Autodesk Fusion 360 part; units mm, degrees
(part 2 of 3)
sketch "b bottom circles" plane through (0, 0, 0) normal (0, 0, 1) x (1, 0, 0) in component "b bottom component"
  line L0 (152.01, 0) -> (302.01, 0)
  line L1 (302.01, 0) -> (302.01, 120)
  line L2 (302.01, 120) -> (152.01, 120)
  line L3 (152.01, 120) -> (152.01, 0)
  circle A0 centre (162.7006, 2.3644) radius 1.005
  circle A1 centre (171.3194, 2.3644) radius 1.005
  circle A2 centre (182.7006, 2.3644) radius 1.005
  circle A3 centre (191.3194, 2.3644) radius 1.005
  circle A4 centre (202.7006, 2.3644) radius 1.005
  circle A5 centre (211.3194, 2.3644) radius 1.005
  circle A6 centre (222.7006, 2.3644) radius 1.005
  circle A7 centre (231.3194, 2.3644) radius 1.005
  circle A8 centre (242.7006, 2.3644) radius 1.005
  circle A9 centre (251.3194, 2.3644) radius 1.005
  circle A10 centre (262.7006, 2.3644) radius 1.005
  circle A11 centre (271.3194, 2.3644) radius 1.005
  circle A12 centre (282.7006, 2.3644) radius 1.005
  circle A13 centre (291.3194, 2.3644) radius 1.005
  circle A14 centre (299.6456, 15.6906) radius 1.005
  circle A15 centre (299.6456, 24.3094) radius 1.005
  circle A16 centre (299.6456, 35.6906) radius 1.005
  circle A17 centre (299.6456, 44.3094) radius 1.005
  circle A18 centre (299.6456, 55.6906) radius 1.005
  circle A19 centre (299.6456, 64.3094) radius 1.005
  circle A20 centre (299.6456, 75.6906) radius 1.005
  circle A21 centre (299.6456, 84.3094) radius 1.005
  circle A22 centre (299.6456, 95.6906) radius 1.005
  circle A23 centre (299.6456, 104.3094) radius 1.005
  circle A24 centre (162.7006, 117.6356) radius 1.005
  circle A25 centre (171.3194, 117.6356) radius 1.005
  circle A26 centre (182.7006, 117.6356) radius 1.005
  circle A27 centre (191.3194, 117.6356) radius 1.005
  circle A28 centre (202.7006, 117.6356) radius 1.005
  circle A29 centre (211.3194, 117.6356) radius 1.005
  circle A30 centre (222.7006, 117.6356) radius 1.005
  circle A31 centre (231.3194, 117.6356) radius 1.005
  circle A32 centre (242.7006, 117.6356) radius 1.005
  circle A33 centre (251.3194, 117.6356) radius 1.005
  circle A34 centre (262.7006, 117.6356) radius 1.005
  circle A35 centre (271.3194, 117.6356) radius 1.005
  circle A36 centre (282.7006, 117.6356) radius 1.005
  circle A37 centre (291.3194, 117.6356) radius 1.005
  circle A38 centre (154.3744, 15.6906) radius 1.005
  circle A39 centre (154.3744, 24.3094) radius 1.005
  circle A40 centre (154.3744, 35.6906) radius 1.005
  circle A41 centre (154.3744, 44.3094) radius 1.005
  circle A42 centre (154.3744, 55.6906) radius 1.005
  circle A43 centre (154.3744, 64.3094) radius 1.005
  circle A44 centre (154.3744, 75.6906) radius 1.005
  circle A45 centre (154.3744, 84.3094) radius 1.005
  circle A46 centre (154.3744, 95.6906) radius 1.005
  circle A47 centre (154.3744, 104.3094) radius 1.005
  dimension "d1612" = 2.01
  dimension "d1613" = 2.01
  dimension "d1614" = 2.01
  dimension "d1615" = 2.01
  dimension "d1616" = 2.01
  dimension "d1617" = 2.01
  dimension "d1618" = 2.01
  dimension "d1619" = 2.01
  dimension "d1620" = 2.01
  dimension "d1621" = 2.01
  dimension "d1622" = 2.01
  dimension "d1623" = 2.01
  dimension "d1624" = 2.01
  dimension "d1625" = 2.01
  dimension "d1647" = 2.01
  dimension "d1648" = 2.01
  dimension "d1649" = 2.01
  dimension "d1650" = 2.01
  dimension "d1651" = 2.01
  dimension "d1652" = 2.01
  dimension "d1653" = 2.01
  dimension "d1654" = 2.01
  dimension "d1655" = 2.01
  dimension "d1656" = 2.01
  dimension "d1686" = 2.01
  dimension "d1687" = 2.01
  dimension "d1688" = 2.01
  dimension "d1689" = 2.01
  dimension "d1690" = 2.01
  dimension "d1691" = 2.01
  dimension "d1692" = 2.01
  dimension "d1693" = 2.01
  dimension "d1694" = 2.01
  dimension "d1695" = 2.01
  dimension "d1696" = 2.01
  dimension "d1697" = 2.01
  dimension "d1698" = 2.01
  dimension "d1699" = 2.01
  dimension "d1721" = 2.01
  dimension "d1722" = 2.01
  dimension "d1723" = 2.01
  dimension "d1724" = 2.01
  dimension "d1725" = 2.01
  dimension "d1726" = 2.01
  dimension "d1727" = 2.01
  dimension "d1728" = 2.01
  dimension "d1729" = 2.01
  dimension "d1730" = 2.01
  measures "d1612" diameter of A0
  measures "d1613" diameter of A1
  measures "d1614" diameter of A2
  measures "d1615" diameter of A3
  measures "d1616" diameter of A4
  measures "d1617" diameter of A5
  measures "d1618" diameter of A6
  measures "d1619" diameter of A7
  measures "d1620" diameter of A8
  measures "d1621" diameter of A9
  measures "d1622" diameter of A10
  measures "d1623" diameter of A11
  measures "d1624" diameter of A12
  measures "d1625" diameter of A13
  measures "d1647" diameter of A14
  measures "d1648" diameter of A15
  measures "d1649" diameter of A16
  measures "d1650" diameter of A17
  measures "d1651" diameter of A18
  measures "d1652" diameter of A19
  measures "d1653" diameter of A20
  measures "d1654" diameter of A21
  measures "d1655" diameter of A22
  measures "d1656" diameter of A23
  measures "d1686" diameter of A24
  measures "d1687" diameter of A25
  measures "d1688" diameter of A26
  measures "d1689" diameter of A27
  measures "d1690" diameter of A28
  measures "d1691" diameter of A29
  measures "d1692" diameter of A30
  measures "d1693" diameter of A31
  measures "d1694" diameter of A32
  measures "d1695" diameter of A33
  measures "d1696" diameter of A34
  measures "d1697" diameter of A35
  measures "d1698" diameter of A36
  measures "d1699" diameter of A37
  measures "d1721" diameter of A38
  measures "d1722" diameter of A39
  measures "d1723" diameter of A40
  measures "d1724" diameter of A41
  measures "d1725" diameter of A42
  measures "d1726" diameter of A43
  measures "d1727" diameter of A44
  measures "d1728" diameter of A45
  measures "d1729" diameter of A46
  measures "d1730" diameter of A47
extrude "b bottom lines body extrude" add sketch "b bottom lines" along normal blind 3.175 separate body makes body 4 in component "b bottom component"
extrude "b bottom circles extrude" add sketch "b bottom circles" along normal blind 3.175 separate body makes body 5 in component "b bottom component"
combine "b bottom lines final combine feature" operation intersect target body 4 tool bodies 5 in component "b bottom component"
sketch "b front lines" plane through (0, 0, 0) normal (0, 0, 1) x (1, 0, 0) in component "b front component"
  line L0 (3.175, 125.185) -> (9.9, 125.185)
  line L1 (9.9, 125.185) -> (9.9, 122.01)
  line L2 (9.9, 122.01) -> (20.1, 122.01)
  line L3 (20.1, 122.01) -> (20.1, 125.185)
  line L4 (20.1, 125.185) -> (29.9, 125.185)
  line L5 (29.9, 125.185) -> (29.9, 122.01)
  line L6 (29.9, 122.01) -> (40.1, 122.01)
  line L7 (40.1, 122.01) -> (40.1, 125.185)
  line L8 (40.1, 125.185) -> (46.825, 125.185)
  line L9 (46.825, 125.185) -> (46.825, 131.91)
  line L10 (46.825, 131.91) -> (50, 131.91)
  line L11 (50, 131.91) -> (50, 142.11)
  line L12 (50, 142.11) -> (46.825, 142.11)
  line L13 (46.825, 142.11) -> (46.825, 151.91)
  line L14 (46.825, 151.91) -> (50, 151.91)
  line L15 (50, 151.91) -> (50, 162.11)
  line L16 (50, 162.11) -> (46.825, 162.11)
  line L17 (46.825, 162.11) -> (46.825, 171.91)
  line L18 (46.825, 171.91) -> (50, 171.91)
  line L19 (50, 171.91) -> (50, 182.11)
  line L20 (50, 182.11) -> (46.825, 182.11)
  line L21 (46.825, 182.11) -> (46.825, 191.91)
  line L22 (46.825, 191.91) -> (50, 191.91)
  line L23 (50, 191.91) -> (50, 202.11)
  line L24 (50, 202.11) -> (46.825, 202.11)
  line L25 (46.825, 202.11) -> (46.825, 211.91)
  line L26 (46.825, 211.91) -> (50, 211.91)
  line L27 (50, 211.91) -> (50, 222.11)
  line L28 (50, 222.11) -> (46.825, 222.11)
  line L29 (46.825, 222.11) -> (46.825, 231.91)
  line L30 (46.825, 231.91) -> (50, 231.91)
  line L31 (50, 231.91) -> (50, 242.11)
  line L32 (50, 242.11) -> (46.825, 242.11)
  line L33 (46.825, 242.11) -> (46.825, 251.91)
  line L34 (46.825, 251.91) -> (50, 251.91)
  line L35 (50, 251.91) -> (50, 262.11)
  line L36 (50, 262.11) -> (46.825, 262.11)
  line L37 (46.825, 262.11) -> (46.825, 268.835)
  line L38 (3.175, 268.835) -> (9.9, 268.835)
  line L39 (9.9, 268.835) -> (9.9, 272.01)
  line L40 (9.9, 272.01) -> (20.1, 272.01)
  line L41 (20.1, 272.01) -> (20.1, 268.835)
  line L42 (20.1, 268.835) -> (29.9, 268.835)
  line L43 (29.9, 268.835) -> (29.9, 272.01)
  line L44 (29.9, 272.01) -> (40.1, 272.01)
  line L45 (40.1, 272.01) -> (40.1, 268.835)
  line L46 (40.1, 268.835) -> (46.825, 268.835)
  line L47 (3.175, 125.185) -> (3.175, 131.91)
  line L48 (3.175, 131.91) -> (0, 131.91)
  line L49 (0, 131.91) -> (0, 142.11)
  line L50 (0, 142.11) -> (3.175, 142.11)
  line L51 (3.175, 142.11) -> (3.175, 151.91)
  line L52 (3.175, 151.91) -> (0, 151.91)
  line L53 (0, 151.91) -> (0, 162.11)
  line L54 (0, 162.11) -> (3.175, 162.11)
  line L55 (3.175, 162.11) -> (3.175, 171.91)
  line L56 (3.175, 171.91) -> (0, 171.91)
  line L57 (0, 171.91) -> (0, 182.11)
  line L58 (0, 182.11) -> (3.175, 182.11)
  line L59 (3.175, 182.11) -> (3.175, 191.91)
  line L60 (3.175, 191.91) -> (0, 191.91)
  line L61 (0, 191.91) -> (0, 202.11)
  line L62 (0, 202.11) -> (3.175, 202.11)
  line L63 (3.175, 202.11) -> (3.175, 211.91)
  line L64 (3.175, 211.91) -> (0, 211.91)
  line L65 (0, 211.91) -> (0, 222.11)
  line L66 (0, 222.11) -> (3.175, 222.11)
  line L67 (3.175, 222.11) -> (3.175, 231.91)
  line L68 (3.175, 231.91) -> (0, 231.91)
  line L69 (0, 231.91) -> (0, 242.11)
  line L70 (0, 242.11) -> (3.175, 242.11)
  line L71 (3.175, 242.11) -> (3.175, 251.91)
  line L72 (3.175, 251.91) -> (0, 251.91)
  line L73 (0, 251.91) -> (0, 262.11)
  line L74 (0, 262.11) -> (3.175, 262.11)
  line L75 (3.175, 262.11) -> (3.175, 268.835)
  dimension "d1735" = 6.725
  dimension "d1736" = 3.175
  dimension "d1737" = 10.2
  dimension "d1738" = 3.175
  dimension "d1739" = 9.8
  dimension "d1740" = 3.175
  dimension "d1741" = 10.2
  dimension "d1742" = 3.175
  dimension "d1743" = 6.725
  dimension "d1748" = 6.725
  dimension "d1749" = 3.175
  dimension "d1750" = 10.2
  dimension "d1751" = 3.175
  dimension "d1752" = 9.8
  dimension "d1753" = 3.175
  dimension "d1754" = 10.2
  dimension "d1755" = 3.175
  dimension "d1756" = 9.8
  dimension "d1757" = 3.175
  dimension "d1758" = 10.2
  dimension "d1759" = 3.175
  dimension "d1760" = 9.8
  dimension "d1761" = 3.175
  dimension "d1762" = 10.2
  dimension "d1763" = 3.175
  dimension "d1764" = 9.8
  dimension "d1765" = 3.175
  dimension "d1766" = 10.2
  dimension "d1767" = 3.175
  dimension "d1768" = 9.8
  dimension "d1769" = 3.175
  dimension "d1770" = 10.2
  dimension "d1771" = 3.175
  dimension "d1772" = 9.8
  dimension "d1773" = 3.175
  dimension "d1774" = 10.2
  dimension "d1775" = 3.175
  dimension "d1776" = 6.725
  dimension "d1791" = 6.725
  dimension "d1792" = 3.175
  dimension "d1793" = 10.2
  dimension "d1794" = 3.175
  dimension "d1795" = 9.8
  dimension "d1796" = 3.175
  dimension "d1797" = 10.2
  dimension "d1798" = 3.175
  dimension "d1799" = 6.725
  dimension "d1804" = 6.725
  dimension "d1805" = 3.175
  dimension "d1806" = 10.2
  dimension "d1807" = 3.175
  dimension "d1808" = 9.8
  dimension "d1809" = 3.175
  dimension "d1810" = 10.2
  dimension "d1811" = 3.175
  dimension "d1812" = 9.8
  dimension "d1813" = 3.175
  dimension "d1814" = 10.2
  dimension "d1815" = 3.175
  dimension "d1816" = 9.8
  dimension "d1817" = 3.175
  dimension "d1818" = 10.2
  dimension "d1819" = 3.175
  dimension "d1820" = 9.8
  dimension "d1821" = 3.175
  dimension "d1822" = 10.2
  dimension "d1823" = 3.175
  dimension "d1824" = 9.8
  dimension "d1825" = 3.175
  dimension "d1826" = 10.2
  dimension "d1827" = 3.175
  dimension "d1828" = 9.8
  dimension "d1829" = 3.175
  dimension "d1830" = 10.2
  dimension "d1831" = 3.175
  dimension "d1832" = 6.725
  constraint horizontal L0
  constraint vertical L1
  constraint horizontal L2
  constraint vertical L3
  constraint horizontal L4
  constraint vertical L5
  constraint horizontal L6
  constraint vertical L7
  constraint horizontal L8
  constraint vertical L9
  constraint horizontal L10
  constraint vertical L11
  constraint horizontal L12
  constraint vertical L13
  constraint horizontal L14
  constraint vertical L15
  constraint horizontal L16
  constraint vertical L17
  constraint horizontal L18
  constraint vertical L19
  constraint horizontal L20
  constraint vertical L21
  constraint horizontal L22
  constraint vertical L23
  constraint horizontal L24
  constraint vertical L25
  constraint horizontal L26
  constraint vertical L27
  constraint horizontal L28
  constraint vertical L29
  constraint horizontal L30
  constraint vertical L31
  constraint horizontal L32
  constraint vertical L33
  constraint horizontal L34
  constraint vertical L35
  constraint horizontal L36
  constraint vertical L37
  constraint horizontal L38
  constraint vertical L39
  constraint horizontal L40
  constraint vertical L41
  constraint horizontal L42
  constraint vertical L43
  constraint horizontal L44
  constraint vertical L45
  constraint horizontal L46
  constraint vertical L47
  constraint horizontal L48
  constraint vertical L49
  constraint horizontal L50
  constraint vertical L51
  constraint horizontal L52
  constraint vertical L53
  constraint horizontal L54
  constraint vertical L55
  constraint horizontal L56
  constraint vertical L57
  constraint horizontal L58
  constraint vertical L59
  constraint horizontal L60
  constraint vertical L61
  constraint horizontal L62
  constraint vertical L63
  constraint horizontal L64
  constraint vertical L65
  constraint horizontal L66
  constraint vertical L67
  constraint horizontal L68
  constraint vertical L69
  constraint horizontal L70
  constraint vertical L71
  constraint horizontal L72
  constraint vertical L73
  constraint horizontal L74
  constraint vertical L75
  measures "d1735" distance of L0.start L0.end
  measures "d1736" distance of L0.end L1.end
  measures "d1737" distance of L1.end L2.end
  measures "d1738" distance of L2.end L3.end
  measures "d1739" distance of L3.end L4.end
  measures "d1740" distance of L4.end L5.end
  measures "d1741" distance of L5.end L6.end
  measures "d1742" distance of L6.end L7.end
  measures "d1743" distance of L7.end L8.end
  measures "d1748" distance of L8.end L9.end
  measures "d1749" distance of L9.end L10.end
  measures "d1750" distance of L10.end L11.end
  measures "d1751" distance of L11.end L12.end
  measures "d1752" distance of L12.end L13.end
  measures "d1753" distance of L13.end L14.end
  measures "d1754" distance of L14.end L15.end
  measures "d1755" distance of L15.end L16.end
  measures "d1756" distance of L16.end L17.end
  measures "d1757" distance of L17.end L18.end
  measures "d1758" distance of L18.end L19.end
  measures "d1759" distance of L19.end L20.end
  measures "d1760" distance of L20.end L21.end
  measures "d1761" distance of L21.end L22.end
  measures "d1762" distance of L22.end L23.end
  measures "d1763" distance of L23.end L24.end
  measures "d1764" distance of L24.end L25.end
  measures "d1765" distance of L25.end L26.end
  measures "d1766" distance of L26.end L27.end
  measures "d1767" distance of L27.end L28.end
  measures "d1768" distance of L28.end L29.end
  measures "d1769" distance of L29.end L30.end
  measures "d1770" distance of L30.end L31.end
  measures "d1771" distance of L31.end L32.end
  measures "d1772" distance of L32.end L33.end
  measures "d1773" distance of L33.end L34.end
  measures "d1774" distance of L34.end L35.end
  measures "d1775" distance of L35.end L36.end
  measures "d1776" distance of L36.end L37.end
  measures "d1791" distance of L38.start L38.end
  measures "d1792" distance of L38.end L39.end
  measures "d1793" distance of L39.end L40.end
  measures "d1794" distance of L40.end L41.end
  measures "d1795" distance of L41.end L42.end
  measures "d1796" distance of L42.end L43.end
  measures "d1797" distance of L43.end L44.end
  measures "d1798" distance of L44.end L45.end
  measures "d1799" distance of L37.end L45.end
  measures "d1804" distance of L0.start L47.end
  measures "d1805" distance of L47.end L48.end
  measures "d1806" distance of L48.end L49.end
  measures "d1807" distance of L49.end L50.end
  measures "d1808" distance of L50.end L51.end
  measures "d1809" distance of L51.end L52.end
  measures "d1810" distance of L52.end L53.end
  measures "d1811" distance of L53.end L54.end
  measures "d1812" distance of L54.end L55.end
  measures "d1813" distance of L55.end L56.end
  measures "d1814" distance of L56.end L57.end
  measures "d1815" distance of L57.end L58.end
  measures "d1816" distance of L58.end L59.end
  measures "d1817" distance of L59.end L60.end
  measures "d1818" distance of L60.end L61.end
  measures "d1819" distance of L61.end L62.end
  measures "d1820" distance of L62.end L63.end
  measures "d1821" distance of L63.end L64.end
  measures "d1822" distance of L64.end L65.end
  measures "d1823" distance of L65.end L66.end
  measures "d1824" distance of L66.end L67.end
  measures "d1825" distance of L67.end L68.end
  measures "d1826" distance of L68.end L69.end
  measures "d1827" distance of L69.end L70.end
  measures "d1828" distance of L70.end L71.end
  measures "d1829" distance of L71.end L72.end
  measures "d1830" distance of L72.end L73.end
  measures "d1831" distance of L73.end L74.end
  measures "d1832" distance of L38.start L74.end
sketch "b front circles" plane through (0, 0, 0) normal (0, 0, 1) x (1, 0, 0) in component "b front component"
  line L0 (0, 122.01) -> (50, 122.01)
  line L1 (50, 122.01) -> (50, 272.01)
  line L2 (50, 272.01) -> (0, 272.01)
  line L3 (0, 272.01) -> (0, 122.01)
  circle A0 centre (9.3094, 124.3744) radius 1.005
  circle A1 centre (20.6906, 124.3744) radius 1.005
  circle A2 centre (29.3094, 124.3744) radius 1.005
  circle A3 centre (40.6906, 124.3744) radius 1.005
  circle A4 centre (47.6356, 131.3194) radius 1.005
  circle A5 centre (47.6356, 142.7006) radius 1.005
  circle A6 centre (47.6356, 151.3194) radius 1.005
  circle A7 centre (47.6356, 162.7006) radius 1.005
  circle A8 centre (47.6356, 171.3194) radius 1.005
  circle A9 centre (47.6356, 182.7006) radius 1.005
  circle A10 centre (47.6356, 191.3194) radius 1.005
  circle A11 centre (47.6356, 202.7006) radius 1.005
  circle A12 centre (47.6356, 211.3194) radius 1.005
  circle A13 centre (47.6356, 222.7006) radius 1.005
  circle A14 centre (47.6356, 231.3194) radius 1.005
  circle A15 centre (47.6356, 242.7006) radius 1.005
  circle A16 centre (47.6356, 251.3194) radius 1.005
  circle A17 centre (47.6356, 262.7006) radius 1.005
  circle A18 centre (9.3094, 269.6456) radius 1.005
  circle A19 centre (20.6906, 269.6456) radius 1.005
  circle A20 centre (29.3094, 269.6456) radius 1.005
  circle A21 centre (40.6906, 269.6456) radius 1.005
  circle A22 centre (2.3644, 131.3194) radius 1.005
  circle A23 centre (2.3644, 142.7006) radius 1.005
  circle A24 centre (2.3644, 151.3194) radius 1.005
  circle A25 centre (2.3644, 162.7006) radius 1.005
  circle A26 centre (2.3644, 171.3194) radius 1.005
  circle A27 centre (2.3644, 182.7006) radius 1.005
  circle A28 centre (2.3644, 191.3194) radius 1.005
  circle A29 centre (2.3644, 202.7006) radius 1.005
  circle A30 centre (2.3644, 211.3194) radius 1.005
  circle A31 centre (2.3644, 222.7006) radius 1.005
  circle A32 centre (2.3644, 231.3194) radius 1.005
  circle A33 centre (2.3644, 242.7006) radius 1.005
  circle A34 centre (2.3644, 251.3194) radius 1.005
  circle A35 centre (2.3644, 262.7006) radius 1.005
  dimension "d1744" = 2.01
  dimension "d1745" = 2.01
  dimension "d1746" = 2.01
  dimension "d1747" = 2.01
  dimension "d1777" = 2.01
  dimension "d1778" = 2.01
  dimension "d1779" = 2.01
  dimension "d1780" = 2.01
  dimension "d1781" = 2.01
  dimension "d1782" = 2.01
  dimension "d1783" = 2.01
  dimension "d1784" = 2.01
  dimension "d1785" = 2.01
  dimension "d1786" = 2.01
  dimension "d1787" = 2.01
  dimension "d1788" = 2.01
  dimension "d1789" = 2.01
  dimension "d1790" = 2.01
  dimension "d1800" = 2.01
  dimension "d1801" = 2.01
  dimension "d1802" = 2.01
  dimension "d1803" = 2.01
  dimension "d1833" = 2.01
  dimension "d1834" = 2.01
  dimension "d1835" = 2.01
  dimension "d1836" = 2.01
  dimension "d1837" = 2.01
  dimension "d1838" = 2.01
  dimension "d1839" = 2.01
  dimension "d1840" = 2.01
  dimension "d1841" = 2.01
  dimension "d1842" = 2.01
  dimension "d1843" = 2.01
  dimension "d1844" = 2.01
  dimension "d1845" = 2.01
  dimension "d1846" = 2.01
  measures "d1744" diameter of A0
  measures "d1745" diameter of A1
  measures "d1746" diameter of A2
  measures "d1747" diameter of A3
  measures "d1777" diameter of A4
  measures "d1778" diameter of A5
  measures "d1779" diameter of A6
  measures "d1780" diameter of A7
  measures "d1781" diameter of A8
  measures "d1782" diameter of A9
  measures "d1783" diameter of A10
  measures "d1784" diameter of A11
  measures "d1785" diameter of A12
  measures "d1786" diameter of A13
  measures "d1787" diameter of A14
  measures "d1788" diameter of A15
  measures "d1789" diameter of A16
  measures "d1790" diameter of A17
  measures "d1800" diameter of A18
  measures "d1801" diameter of A19
  measures "d1802" diameter of A20
  measures "d1803" diameter of A21
  measures "d1833" diameter of A22
  measures "d1834" diameter of A23
  measures "d1835" diameter of A24
  measures "d1836" diameter of A25
  measures "d1837" diameter of A26
  measures "d1838" diameter of A27
  measures "d1839" diameter of A28
  measures "d1840" diameter of A29
  measures "d1841" diameter of A30
  measures "d1842" diameter of A31
  measures "d1843" diameter of A32
  measures "d1844" diameter of A33
  measures "d1845" diameter of A34
  measures "d1846" diameter of A35
extrude "b front lines body extrude" add sketch "b front lines" along normal blind 3.175 separate body makes body 6 in component "b front component"
extrude "b front circles extrude" add sketch "b front circles" along normal blind 3.175 separate body makes body 7 in component "b front component"
combine "b front lines final combine feature" operation intersect target body 6 tool bodies 7 in component "b front component"
sketch "b back lines" plane through (0, 0, 0) normal (0, 0, 1) x (1, 0, 0) in component "b back component"
  line L0 (55.185, 125.185) -> (61.91, 125.185)
  line L1 (61.91, 125.185) -> (61.91, 122.01)
  line L2 (61.91, 122.01) -> (72.11, 122.01)
  line L3 (72.11, 122.01) -> (72.11, 125.185)
  line L4 (72.11, 125.185) -> (81.91, 125.185)
  line L5 (81.91, 125.185) -> (81.91, 122.01)
  line L6 (81.91, 122.01) -> (92.11, 122.01)
  line L7 (92.11, 122.01) -> (92.11, 125.185)
  line L8 (92.11, 125.185) -> (98.835, 125.185)
  line L9 (98.835, 125.185) -> (98.835, 131.91)
  line L10 (98.835, 131.91) -> (102.01, 131.91)
  line L11 (102.01, 131.91) -> (102.01, 142.11)
  line L12 (102.01, 142.11) -> (98.835, 142.11)
  line L13 (98.835, 142.11) -> (98.835, 151.91)
  line L14 (98.835, 151.91) -> (102.01, 151.91)
  line L15 (102.01, 151.91) -> (102.01, 162.11)
  line L16 (102.01, 162.11) -> (98.835, 162.11)
  line L17 (98.835, 162.11) -> (98.835, 171.91)
  line L18 (98.835, 171.91) -> (102.01, 171.91)
  line L19 (102.01, 171.91) -> (102.01, 182.11)
  line L20 (102.01, 182.11) -> (98.835, 182.11)
  line L21 (98.835, 182.11) -> (98.835, 191.91)
  line L22 (98.835, 191.91) -> (102.01, 191.91)
  line L23 (102.01, 191.91) -> (102.01, 202.11)
  line L24 (102.01, 202.11) -> (98.835, 202.11)
  line L25 (98.835, 202.11) -> (98.835, 211.91)
  line L26 (98.835, 211.91) -> (102.01, 211.91)
  line L27 (102.01, 211.91) -> (102.01, 222.11)
  line L28 (102.01, 222.11) -> (98.835, 222.11)
  line L29 (98.835, 222.11) -> (98.835, 231.91)
  line L30 (98.835, 231.91) -> (102.01, 231.91)
  line L31 (102.01, 231.91) -> (102.01, 242.11)
  line L32 (102.01, 242.11) -> (98.835, 242.11)
  line L33 (98.835, 242.11) -> (98.835, 251.91)
  line L34 (98.835, 251.91) -> (102.01, 251.91)
  line L35 (102.01, 251.91) -> (102.01, 262.11)
  line L36 (102.01, 262.11) -> (98.835, 262.11)
  line L37 (98.835, 262.11) -> (98.835, 268.835)
  line L38 (55.185, 268.835) -> (61.91, 268.835)
  line L39 (61.91, 268.835) -> (61.91, 272.01)
  line L40 (61.91, 272.01) -> (72.11, 272.01)
  line L41 (72.11, 272.01) -> (72.11, 268.835)
  line L42 (72.11, 268.835) -> (81.91, 268.835)
  line L43 (81.91, 268.835) -> (81.91, 272.01)
  line L44 (81.91, 272.01) -> (92.11, 272.01)
  line L45 (92.11, 272.01) -> (92.11, 268.835)
  line L46 (92.11, 268.835) -> (98.835, 268.835)
  line L47 (55.185, 125.185) -> (55.185, 131.91)
  line L48 (55.185, 131.91) -> (52.01, 131.91)
  line L49 (52.01, 131.91) -> (52.01, 142.11)
  line L50 (52.01, 142.11) -> (55.185, 142.11)
  line L51 (55.185, 142.11) -> (55.185, 151.91)
  line L52 (55.185, 151.91) -> (52.01, 151.91)
  line L53 (52.01, 151.91) -> (52.01, 162.11)
  line L54 (52.01, 162.11) -> (55.185, 162.11)
  line L55 (55.185, 162.11) -> (55.185, 171.91)
  line L56 (55.185, 171.91) -> (52.01, 171.91)
  line L57 (52.01, 171.91) -> (52.01, 182.11)
  line L58 (52.01, 182.11) -> (55.185, 182.11)
  line L59 (55.185, 182.11) -> (55.185, 191.91)
  line L60 (55.185, 191.91) -> (52.01, 191.91)
  line L61 (52.01, 191.91) -> (52.01, 202.11)
  line L62 (52.01, 202.11) -> (55.185, 202.11)
  line L63 (55.185, 202.11) -> (55.185, 211.91)
  line L64 (55.185, 211.91) -> (52.01, 211.91)
  line L65 (52.01, 211.91) -> (52.01, 222.11)
  line L66 (52.01, 222.11) -> (55.185, 222.11)
  line L67 (55.185, 222.11) -> (55.185, 231.91)
  line L68 (55.185, 231.91) -> (52.01, 231.91)
  line L69 (52.01, 231.91) -> (52.01, 242.11)
  line L70 (52.01, 242.11) -> (55.185, 242.11)
  line L71 (55.185, 242.11) -> (55.185, 251.91)
  line L72 (55.185, 251.91) -> (52.01, 251.91)
  line L73 (52.01, 251.91) -> (52.01, 262.11)
  line L74 (52.01, 262.11) -> (55.185, 262.11)
  line L75 (55.185, 262.11) -> (55.185, 268.835)
  dimension "d1851" = 6.725
  dimension "d1852" = 3.175
  dimension "d1853" = 10.2
  dimension "d1854" = 3.175
  dimension "d1855" = 9.8
  dimension "d1856" = 3.175
  dimension "d1857" = 10.2
  dimension "d1858" = 3.175
  dimension "d1859" = 6.725
  dimension "d1864" = 6.725
  dimension "d1865" = 3.175
  dimension "d1866" = 10.2
  dimension "d1867" = 3.175
  dimension "d1868" = 9.8
  dimension "d1869" = 3.175
  dimension "d1870" = 10.2
  dimension "d1871" = 3.175
  dimension "d1872" = 9.8
  dimension "d1873" = 3.175
  dimension "d1874" = 10.2
  dimension "d1875" = 3.175
  dimension "d1876" = 9.8
  dimension "d1877" = 3.175
  dimension "d1878" = 10.2
  dimension "d1879" = 3.175
  dimension "d1880" = 9.8
  dimension "d1881" = 3.175
  dimension "d1882" = 10.2
  dimension "d1883" = 3.175
  dimension "d1884" = 9.8
  dimension "d1885" = 3.175
  dimension "d1886" = 10.2
  dimension "d1887" = 3.175
  dimension "d1888" = 9.8
  dimension "d1889" = 3.175
  dimension "d1890" = 10.2
  dimension "d1891" = 3.175
  dimension "d1892" = 6.725
  dimension "d1907" = 6.725
  dimension "d1908" = 3.175
  dimension "d1909" = 10.2
  dimension "d1910" = 3.175
  dimension "d1911" = 9.8
  dimension "d1912" = 3.175
  dimension "d1913" = 10.2
  dimension "d1914" = 3.175
  dimension "d1915" = 6.725
  dimension "d1920" = 6.725
  dimension "d1921" = 3.175
  dimension "d1922" = 10.2
  dimension "d1923" = 3.175
  dimension "d1924" = 9.8
  dimension "d1925" = 3.175
  dimension "d1926" = 10.2
  dimension "d1927" = 3.175
  dimension "d1928" = 9.8
  dimension "d1929" = 3.175
  dimension "d1930" = 10.2
  dimension "d1931" = 3.175
  dimension "d1932" = 9.8
  dimension "d1933" = 3.175
  dimension "d1934" = 10.2
  dimension "d1935" = 3.175
  dimension "d1936" = 9.8
  dimension "d1937" = 3.175
  dimension "d1938" = 10.2
  dimension "d1939" = 3.175
  dimension "d1940" = 9.8
  dimension "d1941" = 3.175
  dimension "d1942" = 10.2
  dimension "d1943" = 3.175
  dimension "d1944" = 9.8
  dimension "d1945" = 3.175
  dimension "d1946" = 10.2
  dimension "d1947" = 3.175
  dimension "d1948" = 6.725
  constraint horizontal L0
  constraint vertical L1
  constraint horizontal L2
  constraint vertical L3
  constraint horizontal L4
  constraint vertical L5
  constraint horizontal L6
  constraint vertical L7
  constraint horizontal L8
  constraint vertical L9
  constraint horizontal L10
  constraint vertical L11
  constraint horizontal L12
  constraint vertical L13
  constraint horizontal L14
  constraint vertical L15
  constraint horizontal L16
  constraint vertical L17
  constraint horizontal L18
  constraint vertical L19
  constraint horizontal L20
  constraint vertical L21
  constraint horizontal L22
  constraint vertical L23
  constraint horizontal L24
  constraint vertical L25
  constraint horizontal L26
  constraint vertical L27
  constraint horizontal L28
  constraint vertical L29
  constraint horizontal L30
  constraint vertical L31
  constraint horizontal L32
  constraint vertical L33
  constraint horizontal L34
  constraint vertical L35
  constraint horizontal L36
  constraint vertical L37
  constraint horizontal L38
  constraint vertical L39
  constraint horizontal L40
  constraint vertical L41
  constraint horizontal L42
  constraint vertical L43
  constraint horizontal L44
  constraint vertical L45
  constraint horizontal L46
  constraint vertical L47
  constraint horizontal L48
  constraint vertical L49
  constraint horizontal L50
  constraint vertical L51
  constraint horizontal L52
  constraint vertical L53
  constraint horizontal L54
  constraint vertical L55
  constraint horizontal L56
  constraint vertical L57
  constraint horizontal L58
  constraint vertical L59
  constraint horizontal L60
  constraint vertical L61
  constraint horizontal L62
  constraint vertical L63
  constraint horizontal L64
  constraint vertical L65
  constraint horizontal L66
  constraint vertical L67
  constraint horizontal L68
  constraint vertical L69
  constraint horizontal L70
  constraint vertical L71
  constraint horizontal L72
  constraint vertical L73
  constraint horizontal L74
  constraint vertical L75
  measures "d1851" distance of L0.start L0.end
  measures "d1852" distance of L0.end L1.end
  measures "d1853" distance of L1.end L2.end
  measures "d1854" distance of L2.end L3.end
  measures "d1855" distance of L3.end L4.end
  measures "d1856" distance of L4.end L5.end
  measures "d1857" distance of L5.end L6.end
  measures "d1858" distance of L6.end L7.end
  measures "d1859" distance of L7.end L8.end
  measures "d1864" distance of L8.end L9.end
  measures "d1865" distance of L9.end L10.end
  measures "d1866" distance of L10.end L11.end
  measures "d1867" distance of L11.end L12.end
  measures "d1868" distance of L12.end L13.end
  measures "d1869" distance of L13.end L14.end
  measures "d1870" distance of L14.end L15.end
  measures "d1871" distance of L15.end L16.end
  measures "d1872" distance of L16.end L17.end
  measures "d1873" distance of L17.end L18.end
  measures "d1874" distance of L18.end L19.end
  measures "d1875" distance of L19.end L20.end
  measures "d1876" distance of L20.end L21.end
  measures "d1877" distance of L21.end L22.end
  measures "d1878" distance of L22.end L23.end
  measures "d1879" distance of L23.end L24.end
  measures "d1880" distance of L24.end L25.end
  measures "d1881" distance of L25.end L26.end
  measures "d1882" distance of L26.end L27.end
  measures "d1883" distance of L27.end L28.end
  measures "d1884" distance of L28.end L29.end
  measures "d1885" distance of L29.end L30.end
  measures "d1886" distance of L30.end L31.end
  measures "d1887" distance of L31.end L32.end
  measures "d1888" distance of L32.end L33.end
  measures "d1889" distance of L33.end L34.end
  measures "d1890" distance of L34.end L35.end
  measures "d1891" distance of L35.end L36.end
  measures "d1892" distance of L36.end L37.end
  measures "d1907" distance of L38.start L38.end
  measures "d1908" distance of L38.end L39.end
  measures "d1909" distance of L39.end L40.end
  measures "d1910" distance of L40.end L41.end
  measures "d1911" distance of L41.end L42.end
  measures "d1912" distance of L42.end L43.end
  measures "d1913" distance of L43.end L44.end
  measures "d1914" distance of L44.end L45.end
  measures "d1915" distance of L37.end L45.end
  measures "d1920" distance of L0.start L47.end
  measures "d1921" distance of L47.end L48.end
  measures "d1922" distance of L48.end L49.end
  measures "d1923" distance of L49.end L50.end
  measures "d1924" distance of L50.end L51.end
  measures "d1925" distance of L51.end L52.end
  measures "d1926" distance of L52.end L53.end
  measures "d1927" distance of L53.end L54.end
  measures "d1928" distance of L54.end L55.end
  measures "d1929" distance of L55.end L56.end
  measures "d1930" distance of L56.end L57.end
  measures "d1931" distance of L57.end L58.end
  measures "d1932" distance of L58.end L59.end
  measures "d1933" distance of L59.end L60.end
  measures "d1934" distance of L60.end L61.end
  measures "d1935" distance of L61.end L62.end
  measures "d1936" distance of L62.end L63.end
  measures "d1937" distance of L63.end L64.end
  measures "d1938" distance of L64.end L65.end
  measures "d1939" distance of L65.end L66.end
  measures "d1940" distance of L66.end L67.end
  measures "d1941" distance of L67.end L68.end
  measures "d1942" distance of L68.end L69.end
  measures "d1943" distance of L69.end L70.end
  measures "d1944" distance of L70.end L71.end
  measures "d1945" distance of L71.end L72.end
  measures "d1946" distance of L72.end L73.end
  measures "d1947" distance of L73.end L74.end
  measures "d1948" distance of L38.start L74.end
sketch "b back circles" plane through (0, 0, 0) normal (0, 0, 1) x (1, 0, 0) in component "b back component"
  line L0 (52.01, 122.01) -> (102.01, 122.01)
  line L1 (102.01, 122.01) -> (102.01, 272.01)
  line L2 (102.01, 272.01) -> (52.01, 272.01)
  line L3 (52.01, 272.01) -> (52.01, 122.01)
  circle A0 centre (61.3194, 124.3744) radius 1.005
  circle A1 centre (72.7006, 124.3744) radius 1.005
  circle A2 centre (81.3194, 124.3744) radius 1.005
  circle A3 centre (92.7006, 124.3744) radius 1.005
  circle A4 centre (99.6456, 131.3194) radius 1.005
  circle A5 centre (99.6456, 142.7006) radius 1.005
  circle A6 centre (99.6456, 151.3194) radius 1.005
  circle A7 centre (99.6456, 162.7006) radius 1.005
  circle A8 centre (99.6456, 171.3194) radius 1.005
  circle A9 centre (99.6456, 182.7006) radius 1.005
  circle A10 centre (99.6456, 191.3194) radius 1.005
  circle A11 centre (99.6456, 202.7006) radius 1.005
  circle A12 centre (99.6456, 211.3194) radius 1.005
  circle A13 centre (99.6456, 222.7006) radius 1.005
  circle A14 centre (99.6456, 231.3194) radius 1.005
  circle A15 centre (99.6456, 242.7006) radius 1.005
  circle A16 centre (99.6456, 251.3194) radius 1.005
  circle A17 centre (99.6456, 262.7006) radius 1.005
  circle A18 centre (61.3194, 269.6456) radius 1.005
  circle A19 centre (72.7006, 269.6456) radius 1.005
  circle A20 centre (81.3194, 269.6456) radius 1.005
  circle A21 centre (92.7006, 269.6456) radius 1.005
  circle A22 centre (54.3744, 131.3194) radius 1.005
  circle A23 centre (54.3744, 142.7006) radius 1.005
  circle A24 centre (54.3744, 151.3194) radius 1.005
  circle A25 centre (54.3744, 162.7006) radius 1.005
  circle A26 centre (54.3744, 171.3194) radius 1.005
  circle A27 centre (54.3744, 182.7006) radius 1.005
  circle A28 centre (54.3744, 191.3194) radius 1.005
  circle A29 centre (54.3744, 202.7006) radius 1.005
  circle A30 centre (54.3744, 211.3194) radius 1.005
  circle A31 centre (54.3744, 222.7006) radius 1.005
  circle A32 centre (54.3744, 231.3194) radius 1.005
  circle A33 centre (54.3744, 242.7006) radius 1.005
  circle A34 centre (54.3744, 251.3194) radius 1.005
  circle A35 centre (54.3744, 262.7006) radius 1.005
  dimension "d1860" = 2.01
  dimension "d1861" = 2.01
  dimension "d1862" = 2.01
  dimension "d1863" = 2.01
  dimension "d1893" = 2.01
  dimension "d1894" = 2.01
  dimension "d1895" = 2.01
  dimension "d1896" = 2.01
  dimension "d1897" = 2.01
  dimension "d1898" = 2.01
  dimension "d1899" = 2.01
  dimension "d1900" = 2.01
  dimension "d1901" = 2.01
  dimension "d1902" = 2.01
  dimension "d1903" = 2.01
  dimension "d1904" = 2.01
  dimension "d1905" = 2.01
  dimension "d1906" = 2.01
  dimension "d1916" = 2.01
  dimension "d1917" = 2.01
  dimension "d1918" = 2.01
  dimension "d1919" = 2.01
  dimension "d1949" = 2.01
  dimension "d1950" = 2.01
  dimension "d1951" = 2.01
  dimension "d1952" = 2.01
  dimension "d1953" = 2.01
  dimension "d1954" = 2.01
  dimension "d1955" = 2.01
  dimension "d1956" = 2.01
  dimension "d1957" = 2.01
  dimension "d1958" = 2.01
  dimension "d1959" = 2.01
  dimension "d1960" = 2.01
  dimension "d1961" = 2.01
  dimension "d1962" = 2.01
  measures "d1860" diameter of A0
  measures "d1861" diameter of A1
  measures "d1862" diameter of A2
  measures "d1863" diameter of A3
  measures "d1893" diameter of A4
  measures "d1894" diameter of A5
  measures "d1895" diameter of A6
  measures "d1896" diameter of A7
  measures "d1897" diameter of A8
  measures "d1898" diameter of A9
  measures "d1899" diameter of A10
  measures "d1900" diameter of A11
  measures "d1901" diameter of A12
  measures "d1902" diameter of A13
  measures "d1903" diameter of A14
  measures "d1904" diameter of A15
  measures "d1905" diameter of A16
  measures "d1906" diameter of A17
  measures "d1916" diameter of A18
  measures "d1917" diameter of A19
  measures "d1918" diameter of A20
  measures "d1919" diameter of A21
  measures "d1949" diameter of A22
  measures "d1950" diameter of A23
  measures "d1951" diameter of A24
  measures "d1952" diameter of A25
  measures "d1953" diameter of A26
  measures "d1954" diameter of A27
  measures "d1955" diameter of A28
  measures "d1956" diameter of A29
  measures "d1957" diameter of A30
  measures "d1958" diameter of A31
  measures "d1959" diameter of A32
  measures "d1960" diameter of A33
  measures "d1961" diameter of A34
  measures "d1962" diameter of A35
extrude "b back lines body extrude" add sketch "b back lines" along normal blind 3.175 separate body makes body 8 in component "b back component"
extrude "b back circles extrude" add sketch "b back circles" along normal blind 3.175 separate body makes body 9 in component "b back component"
combine "b back lines final combine feature" operation intersect target body 8 tool bodies 9 in component "b back component"
sketch "b left lines" plane through (0, 0, 0) normal (0, 0, 1) x (1, 0, 0) in component "b left component"
  line L0 (107.195, 122.01) -> (114.12, 122.01)
  line L1 (114.12, 122.01) -> (114.12, 125.185)
  line L2 (114.12, 125.185) -> (123.92, 125.185)
  line L3 (123.92, 125.185) -> (123.92, 122.01)
  line L4 (123.92, 122.01) -> (134.12, 122.01)
  line L5 (134.12, 122.01) -> (134.12, 125.185)
  line L6 (134.12, 125.185) -> (143.92, 125.185)
  line L7 (143.92, 125.185) -> (143.92, 122.01)
  line L8 (143.92, 122.01) -> (150.845, 122.01)
  line L9 (150.845, 122.01) -> (150.845, 136.91)
  line L10 (150.845, 136.91) -> (154.02, 136.91)
  line L11 (154.02, 136.91) -> (154.02, 147.11)
  line L12 (154.02, 147.11) -> (150.845, 147.11)
  line L13 (150.845, 147.11) -> (150.845, 156.91)
  line L14 (150.845, 156.91) -> (154.02, 156.91)
  line L15 (154.02, 156.91) -> (154.02, 167.11)
  line L16 (154.02, 167.11) -> (150.845, 167.11)
  line L17 (150.845, 167.11) -> (150.845, 176.91)
  line L18 (150.845, 176.91) -> (154.02, 176.91)
  line L19 (154.02, 176.91) -> (154.02, 187.11)
  line L20 (154.02, 187.11) -> (150.845, 187.11)
  line L21 (150.845, 187.11) -> (150.845, 196.91)
  line L22 (150.845, 196.91) -> (154.02, 196.91)
  line L23 (154.02, 196.91) -> (154.02, 207.11)
  line L24 (154.02, 207.11) -> (150.845, 207.11)
  line L25 (150.845, 207.11) -> (150.845, 216.91)
  line L26 (150.845, 216.91) -> (154.02, 216.91)
  line L27 (154.02, 216.91) -> (154.02, 227.11)
  line L28 (154.02, 227.11) -> (150.845, 227.11)
  line L29 (150.845, 227.11) -> (150.845, 242.01)
  line L30 (107.195, 242.01) -> (114.12, 242.01)
  line L31 (114.12, 242.01) -> (114.12, 238.835)
  line L32 (114.12, 238.835) -> (123.92, 238.835)
  line L33 (123.92, 238.835) -> (123.92, 242.01)
  line L34 (123.92, 242.01) -> (134.12, 242.01)
  line L35 (134.12, 242.01) -> (134.12, 238.835)
  line L36 (134.12, 238.835) -> (143.92, 238.835)
  line L37 (143.92, 238.835) -> (143.92, 242.01)
  line L38 (143.92, 242.01) -> (150.845, 242.01)
  line L39 (107.195, 122.01) -> (107.195, 136.91)
  line L40 (107.195, 136.91) -> (104.02, 136.91)
  line L41 (104.02, 136.91) -> (104.02, 147.11)
  line L42 (104.02, 147.11) -> (107.195, 147.11)
  line L43 (107.195, 147.11) -> (107.195, 156.91)
  line L44 (107.195, 156.91) -> (104.02, 156.91)
  line L45 (104.02, 156.91) -> (104.02, 167.11)
  line L46 (104.02, 167.11) -> (107.195, 167.11)
  line L47 (107.195, 167.11) -> (107.195, 176.91)
  line L48 (107.195, 176.91) -> (104.02, 176.91)
  line L49 (104.02, 176.91) -> (104.02, 187.11)
  line L50 (104.02, 187.11) -> (107.195, 187.11)
  line L51 (107.195, 187.11) -> (107.195, 196.91)
  line L52 (107.195, 196.91) -> (104.02, 196.91)
  line L53 (104.02, 196.91) -> (104.02, 207.11)
  line L54 (104.02, 207.11) -> (107.195, 207.11)
  line L55 (107.195, 207.11) -> (107.195, 216.91)
  line L56 (107.195, 216.91) -> (104.02, 216.91)
  line L57 (104.02, 216.91) -> (104.02, 227.11)
  line L58 (104.02, 227.11) -> (107.195, 227.11)
  line L59 (107.195, 227.11) -> (107.195, 242.01)
  dimension "d1967" = 6.925
  dimension "d1968" = 3.175
  dimension "d1969" = 9.8
  dimension "d1970" = 3.175
  dimension "d1971" = 10.2
  dimension "d1972" = 3.175
  dimension "d1973" = 9.8
  dimension "d1974" = 3.175
  dimension "d1975" = 6.925
  dimension "d1980" = 14.9
  dimension "d1981" = 3.175
  dimension "d1982" = 10.2
  dimension "d1983" = 3.175
  dimension "d1984" = 9.8
  dimension "d1985" = 3.175
  dimension "d1986" = 10.2
  dimension "d1987" = 3.175
  dimension "d1988" = 9.8
  dimension "d1989" = 3.175
  dimension "d1990" = 10.2
  dimension "d1991" = 3.175
  dimension "d1992" = 9.8
  dimension "d1993" = 3.175
  dimension "d1994" = 10.2
  dimension "d1995" = 3.175
  dimension "d1996" = 9.8
  dimension "d1997" = 3.175
  dimension "d1998" = 10.2
  dimension "d1999" = 3.175
  dimension "d2000" = 14.9
  dimension "d2011" = 6.925
  dimension "d2012" = 3.175
  dimension "d2013" = 9.8
  dimension "d2014" = 3.175
  dimension "d2015" = 10.2
  dimension "d2016" = 3.175
  dimension "d2017" = 9.8
  dimension "d2018" = 3.175
  dimension "d2019" = 6.925
  dimension "d2024" = 14.9
  dimension "d2025" = 3.175
  dimension "d2026" = 10.2
  dimension "d2027" = 3.175
  dimension "d2028" = 9.8
  dimension "d2029" = 3.175
  dimension "d2030" = 10.2
  dimension "d2031" = 3.175
  dimension "d2032" = 9.8
  dimension "d2033" = 3.175
  dimension "d2034" = 10.2
  dimension "d2035" = 3.175
  dimension "d2036" = 9.8
  dimension "d2037" = 3.175
  dimension "d2038" = 10.2
  dimension "d2039" = 3.175
  dimension "d2040" = 9.8
  dimension "d2041" = 3.175
  dimension "d2042" = 10.2
  dimension "d2043" = 3.175
  dimension "d2044" = 14.9
  constraint horizontal L0
  constraint vertical L1
  constraint horizontal L2
  constraint vertical L3
  constraint horizontal L4
  constraint vertical L5
  constraint horizontal L6
  constraint vertical L7
  constraint horizontal L8
  constraint vertical L9
  constraint horizontal L10
  constraint vertical L11
  constraint horizontal L12
  constraint vertical L13
  constraint horizontal L14
  constraint vertical L15
  constraint horizontal L16
  constraint vertical L17
  constraint horizontal L18
  constraint vertical L19
  constraint horizontal L20
  constraint vertical L21
  constraint horizontal L22
  constraint vertical L23
  constraint horizontal L24
  constraint vertical L25
  constraint horizontal L26
  constraint vertical L27
  constraint horizontal L28
  constraint vertical L29
  constraint horizontal L30
  constraint vertical L31
  constraint horizontal L32
  constraint vertical L33
  constraint horizontal L34
  constraint vertical L35
  constraint horizontal L36
  constraint vertical L37
  constraint horizontal L38
  constraint vertical L39
  constraint horizontal L40
  constraint vertical L41
  constraint horizontal L42
  constraint vertical L43
  constraint horizontal L44
  constraint vertical L45
  constraint horizontal L46
  constraint vertical L47
  constraint horizontal L48
  constraint vertical L49
  constraint horizontal L50
  constraint vertical L51
  constraint horizontal L52
  constraint vertical L53
  constraint horizontal L54
  constraint vertical L55
  constraint horizontal L56
  constraint vertical L57
  constraint horizontal L58
  constraint vertical L59
  measures "d1967" distance of L0.start L0.end
  measures "d1968" distance of L0.end L1.end
  measures "d1969" distance of L1.end L2.end
  measures "d1970" distance of L2.end L3.end
  measures "d1971" distance of L3.end L4.end
  measures "d1972" distance of L4.end L5.end
  measures "d1973" distance of L5.end L6.end
  measures "d1974" distance of L6.end L7.end
  measures "d1975" distance of L7.end L8.end
  measures "d1980" distance of L8.end L9.end
  measures "d1981" distance of L9.end L10.end
  measures "d1982" distance of L10.end L11.end
  measures "d1983" distance of L11.end L12.end
  measures "d1984" distance of L12.end L13.end
  measures "d1985" distance of L13.end L14.end
  measures "d1986" distance of L14.end L15.end
  measures "d1987" distance of L15.end L16.end
  measures "d1988" distance of L16.end L17.end
  measures "d1989" distance of L17.end L18.end
  measures "d1990" distance of L18.end L19.end
  measures "d1991" distance of L19.end L20.end
  measures "d1992" distance of L20.end L21.end
  measures "d1993" distance of L21.end L22.end
  measures "d1994" distance of L22.end L23.end
  measures "d1995" distance of L23.end L24.end
  measures "d1996" distance of L24.end L25.end
  measures "d1997" distance of L25.end L26.end
  measures "d1998" distance of L26.end L27.end
  measures "d1999" distance of L27.end L28.end
  measures "d2000" distance of L28.end L29.end
  measures "d2011" distance of L30.start L30.end
  measures "d2012" distance of L30.end L31.end
  measures "d2013" distance of L31.end L32.end
  measures "d2014" distance of L32.end L33.end
  measures "d2015" distance of L33.end L34.end
  measures "d2016" distance of L34.end L35.end
  measures "d2017" distance of L35.end L36.end
  measures "d2018" distance of L36.end L37.end
  measures "d2019" distance of L29.end L37.end
  measures "d2024" distance of L0.start L39.end
  measures "d2025" distance of L39.end L40.end
  measures "d2026" distance of L40.end L41.end
  measures "d2027" distance of L41.end L42.end
  measures "d2028" distance of L42.end L43.end
  measures "d2029" distance of L43.end L44.end
  measures "d2030" distance of L44.end L45.end
  measures "d2031" distance of L45.end L46.end
  measures "d2032" distance of L46.end L47.end
  measures "d2033" distance of L47.end L48.end
  measures "d2034" distance of L48.end L49.end
  measures "d2035" distance of L49.end L50.end
  measures "d2036" distance of L50.end L51.end
  measures "d2037" distance of L51.end L52.end
  measures "d2038" distance of L52.end L53.end
  measures "d2039" distance of L53.end L54.end
  measures "d2040" distance of L54.end L55.end
  measures "d2041" distance of L55.end L56.end
  measures "d2042" distance of L56.end L57.end
  measures "d2043" distance of L57.end L58.end
  measures "d2044" distance of L30.start L58.end